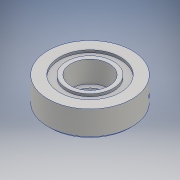
# Autodesk Inventor part: joint_mag_side
Saved by Autodesk Inventor 2017 (Build 210142000, 142)
## iProperties
Created: 2017-09-26
Part Number: joint_mag_side
Material: Aluminum 6061
Document SubType Name: Modeling
Designer: Thoma
Density: 2.7 g/cm^3
Appearance: Aluminum - Flat
Author: Thoma
Autodesk Inventor part; units mm, degrees
sketch "Sketch1" plane through (0, 0, 0) normal (0, 0, 1) x (1, 0, 0)
  circle A0 centre (0, 0) radius 35
  circle A1 centre (0, 0) radius 12
  dimension "d0" = 70
  dimension "d1" = 24
  constraints: 2 centre point, 2 coincident
  measures "d0" diameter of A0
  measures "d1" diameter of A1
extrude "Extrusion1" add sketch "Sketch1" along normal blind 22
sketch "Sketch2" plane through (0, 0, 22) normal (0, 0, 1) x (1, 0, 0)
  circle A0 centre (0, 0) radius 12 projected
  circle A1 centre (0, 0) radius 35 projected
  circle A2 centre (0, 0) radius 25.5
  circle A3 centre (0, 0) radius 19.5
  dimension "d4" = 51
  dimension "d5" = 6
  constraints: 2 centre point, 1 coincident
  measures "d4" diameter of A2
  measures "d5" radial gap between concentric circles of A2 A3
extrude "Extrusion2" cut sketch "Sketch2" against normal blind 2.1 contours A2
sketch "Sketch3" plane through (0, 0, 22) normal (0, 0, 1) x (1, 0, 0)
  line L0 (0, 0) -> (0, 45.779) construction
  line L1 (0, 0) -> (38.81, 0) construction
  line L2 (0, 0) -> (26.8116, 22.4976) construction
  circle A0 centre (0, 0) radius 35 construction
  line L3 (0, 0) -> (35, 0) construction
  line L4 (0, 0) -> (17.5, 30.3109) construction
  line L5 (0, 0) -> (35, 0) construction
  line L6 (0, 0) -> (-26.8116, 22.4976) construction
  line L7 (0, 0) -> (-17.5, 30.3109) construction
  dimension "d11" = 40
  dimension "d12" = 60
  constraints: 16 end point, 3 horizontal, 2 equal length, 2 point on circle, 2 symmetric about line, 1 vertical
  measures "d11" angle of L3 L2
  measures "d12" angle of L5 L4
ref_plane "Work Plane1" through (17.5, 30.3109, 22) normal (0.5, 0.866, 0) x (-0.866, 0.5, 0)
ref_plane "Work Plane2" through (26.8116, 22.4976, 22) normal (0.766, 0.6428, 0) x (-0.6428, 0.766, 0)
ref_plane "Work Plane3" through (-17.5, 30.3109, 22) normal (-0.5, 0.866, 0) x (-0.866, -0.5, 0)
ref_plane "Work Plane4" through (-26.8116, 22.4976, 22) normal (-0.766, 0.6428, 0) x (-0.6428, -0.766, 0)
sketch "Sketch4" plane through (26.8116, 22.4976, 22) normal (0.766, 0.6428, 0) x (-0.6428, 0.766, 0)
  line L0 (35, 0) -> (-35, 0) projected
  point P0 (0, -22)
  point P1 (0, -13)
  dimension "d13" = 13
  measures "d13" distance from line of L0 point (0, -13)
hole "Hole1" at (26.8116, 22.4976, 9) direction (-0.766, -0.6428, 0) diameter 3 depth 4 tip angle 118
sketch "Sketch5" plane through (17.5, 30.3109, 22) normal (0.5, 0.866, 0) x (-0.866, 0.5, 0)
  line L0 (35, 0) -> (-35, 0) projected
  point P0 (0, -22)
  point P1 (0, -13)
  dimension "d21" = 13
  measures "d21" distance from line of L0 point (0, -13)
hole "Hole2" at (17.5, 30.3109, 9) direction (-0.5, -0.866, 0) diameter 3 depth 8 tip angle 118
sketch "Sketch6" plane through (-17.5, 30.3109, 22) normal (-0.5, 0.866, 0) x (-0.866, -0.5, 0)
  line L0 (35, 0) -> (-35, 0) projected
  point P0 (0, -22)
  point P1 (0, -13)
  dimension "d29" = 13
  measures "d29" distance from line of L0 point (0, -13)
hole "Hole3" at (-17.5, 30.3109, 9) direction (0.5, -0.866, 0) diameter 3 depth 8 tip angle 118
sketch "Sketch7" plane through (-26.8116, 22.4976, 22) normal (-0.766, 0.6428, 0) x (-0.6428, -0.766, 0)
  line L0 (35, 0) -> (-35, 0) projected
  point P0 (0, -22)
  point P1 (0, -13)
  dimension "d37" = 13
  measures "d37" distance from line of L0 point (0, -13)
hole "Hole4" at (-26.8116, 22.4976, 9) direction (0.766, -0.6428, 0) diameter 3 depth 8 tip angle 118
thread "Thread1" size "M3x0.5" class "6H" standard "ANSI Metric M Profile" full length
thread "Thread2" size "M3x0.5" class "6H" standard "ANSI Metric M Profile" full length
thread "Thread3" size "M3x0.5" class "6H" standard "ANSI Metric M Profile" full length
thread "Thread4" size "M3x0.5" class "6H" standard "ANSI Metric M Profile" full length
sketch "Sketch9" plane through (0, 0, 22) normal (0, 0, 1) x (1, 0, 0)
  circle A0 centre (0, 0) radius 16
  dimension "d53" = 32
  constraints: 1 centre point, 1 coincident
  measures "d53" diameter of A0
extrude "Extrusion3" cut sketch "Sketch9" against normal blind 18
sketch "Sketch11" plane through (0, 0, 0) normal (0, 0, -1) x (-1, 0, 0)
  circle A0 centre (0, 0) radius 27 construction
  point P0 (-27, 0)
  point P1 (0, -27)
  point P2 (27, 0)
  point P3 (0, 27)
  dimension "d77" = 54
  dimension "d80" = 360
  constraints: 1 coincident, 1 horizontal alignment, 7 other
hole "Hole6" at (27, 0, 0) at (0, -27, 0) at (-27, 0, 0) at (0, 27, 0) direction (0, 0, 1) diameter 3 depth 8 tip angle 118
thread "Thread9" size "M3x0.5" class "6H" standard "ANSI Metric M Profile" full length
thread "Thread10" size "M3x0.5" class "6H" standard "ANSI Metric M Profile" full length
thread "Thread11" size "M3x0.5" class "6H" standard "ANSI Metric M Profile" full length
thread "Thread12" size "M3x0.5" class "6H" standard "ANSI Metric M Profile" full length
chamfer "Chamfer2" distance 2 angle 45 1 edges at (-35, 0, 0)
body "Solid1"
